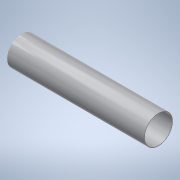
# Autodesk Inventor part: tubo pre distribucion
Saved by Autodesk Inventor 2020 (Build 240168000, 168)
## iProperties
Created: 2020-02-18
Part Number: tubo pre distribucion
Material: PVC, no plastificado
Document SubType Name: Modeling
Designer: PabloGod
Mass: 112.157 g
Surface Area: 1165.04 cm^2
Volume: 86.9436 cm^3
Density: 1.29 g/cm^3
Appearance: Suave - Blanco
Author: PabloGod
Autodesk Inventor part; units mm, degrees
ref_plane "YZ Plane" through (0, 0, 0) normal (1, 0, 0) x (0, 1, 0)
ref_plane "XZ Plane" through (0, 0, 0) normal (0, 1, 0) x (-1, 0, 0)
ref_plane "XY Plane" through (0, 0, 0) normal (0, 0, 1) x (1, 0, 0)
sketch "Boceto1" plane through (0, 0, 0) normal (1, 0, 0) x (0, 1, 0)
  circle A0 centre (0, 0) radius 30
  circle A1 centre (0, 0) radius 31.5
  dimension "d0" = 60
  dimension "d1" = 63
  constraints: 2 centre point, 2 coincident
  measures "d0" diameter of A0
  measures "d1" diameter of A1
extrude "Extrusión1" add sketch "Boceto1" along normal blind 300
